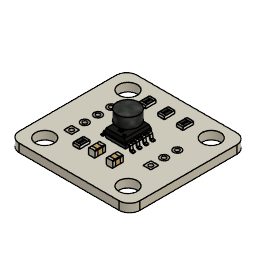
AS5600 Clamp (Autodesk Fusion 360 archive; units mm, degrees)
design "AS5600_magnetic_encoder"
part number: AS5600_magnetic_encoder
Autodesk Fusion 360 part; units mm, degrees
note: some values were not read from the file. Chosen so that the rebuilt part matches the saved one: a direction.
other "DerivedContext1"
imported_body "Base Feature1" makes body 1 makes body 2 makes body 3 makes body 4 makes body 5 makes body 6 makes body 7 makes body 8 makes body 9 makes body 10 makes body 11 makes body 12 makes body 13 makes body 14 makes body 15 makes body 16 makes body 17 makes body 18 makes body 19 makes body 20 makes body 21 makes body 22 makes body 23 makes body 24 makes body 25 makes body 26 makes body 27 makes body 28
sketch "sketch 657" plane through (0, 0, 8.4) normal (0, 0, -1) x (1, 0, 0)
  circle A0 centre (0, 0) radius 1.585
  circle A1 centre (0, 0) radius 2.1
extrude "Extrude1" add sketch "sketch 657" along normal blind 2 from surface at 0.5 separate body contours A0 | A1 makes body 29
copy_body "Body->Comp1" bodies 29 removing the originals makes body 30 in component "Magnet"
move_body "Move1" bodies 30 to x (1, 0, 0) y (0, 1, 0) z (0, 0, 1) at (0, 0, -3) in component "Magnet"
component "Magnet" placed x (1, 0, 0) y (0, 1, 0) z (0, 0, 1) at (0, 0, 0)
named bodies: "Magnet"
